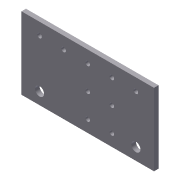
# Autodesk Inventor part: Frame_TopFrontRollerPlate
Saved by Autodesk Inventor 2012 (Build 160160000, 160)
## iProperties
Created: 2012-01-09
Part Number: Frame_TopFrontRollerPlate
Material: Aluminum-6061
Document SubType Name: Modeling
Designer: JesseK
Mass: 133.482 g
Surface Area: 236.674 cm^2
Volume: 49.2552 cm^3
Density: 2.71 g/cm^3
Author: JesseK
Autodesk Inventor part; units mm, degrees
ref_plane "YZ Plane" through (0, 0, 0) normal (1, 0, 0) x (0, 1, 0)
ref_plane "XZ Plane" through (0, 0, 0) normal (0, 1, 0) x (-1, 0, 0)
ref_plane "XY Plane" through (0, 0, 0) normal (0, 0, 1) x (1, 0, 0)
sketch "Sketch1" plane through (0, 0, 0) normal (0, 0, 1) x (1, 0, 0)
  line L0 (0, 0) -> (139.7, 0)
  line L1 (139.7, 0) -> (139.7, 76.2)
  line L2 (139.7, 76.2) -> (0, 76.2)
  line L3 (0, 76.2) -> (0, 0)
  dimension "d0" = 139.7
  dimension "d1" = 76.2
  constraints: 8 end point, 2 parallel, 1 horizontal, 1 perpendicular
  measures "d0" distance between parallel lines of L1 L3
  measures "d1" distance between parallel lines of L0 L2
extrude "Extrusion1" add sketch "Sketch1" along normal blind 4.7625
sketch "Sketch2" plane through (0, 0, 4.7625) normal (0, 0, 1) x (1, 0, 0)
  line L0 (0, 0) -> (0, 76.2) projected
  line L1 (139.7, 0) -> (0, 0) projected
  circle A0 centre (19.05, 12.7) radius 4.7625
  circle A1 centre (120.65, 12.7) radius 4.7625
  line L2 (19.05, 12.7) -> (120.65, 12.7) construction
  dimension "d4" = 12.7
  dimension "d5" = 19.05
  dimension "d6" = 101.6
  dimension "d7" = 9.525
  constraints: 2 centre point, 2 end point, 1 equal radius, 1 horizontal
  measures "d4" distance from line of L1 L2.start
  measures "d5" distance from line of L0 L2.start
  measures "d6" distance of L2.end L2.start
  measures "d7" diameter of A0
extrude "Extrusion2" cut sketch "Sketch2" against normal up to next
sketch "Sketch3" plane through (0, 0, 4.7625) normal (0, 0, 1) x (1, 0, 0)
  circle A0 centre (19.05, 12.7) radius 4.7625 projected
  line L0 (139.7, 0) -> (0, 0) projected
  circle A1 centre (69.85, 12.7) radius 2.3813
  dimension "d10" = 4.7625
  dimension "d11" = 12.7
  dimension "d13" = 50.8
  constraints: 1 centre point
  measures "d10" diameter of A1
  measures "d11" distance from line of L0 A1.centre
  measures "d13" distance of A1.centre A0.centre
extrude "Extrusion3" cut sketch "Sketch3" against normal up to next contours A1
pattern_linear "Rectangular Pattern1" count 2 spacing 25.4 along (0, 1, 0) count 2 spacing 25.4 along (1, 0, 0) of "Extrusion3"
sketch "Sketch4" plane through (0, 0, 4.7625) normal (0, 0, 1) x (1, 0, 0)
  line L0 (0, 0) -> (0, 76.2) projected
  line L1 (0, 76.2) -> (139.7, 76.2) projected
  circle A0 centre (19.05, 63.5) radius 2.3813
  dimension "d22" = 4.7625
  dimension "d23" = 12.7
  dimension "d24" = 19.05
  constraints: 1 centre point
  measures "d22" diameter of A0
  measures "d23" distance from line of L1 A0.centre
  measures "d24" distance from line of L0 A0.centre
extrude "Extrusion4" cut sketch "Sketch4" against normal up to next
pattern_linear "Rectangular Pattern2" count 5 spacing 25.4 along (1, 0, 0) of "Extrusion4"
body "Solid1"
